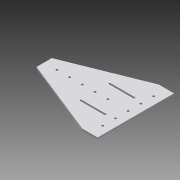
# Autodesk Inventor part: traingle_bracket(tb)
Saved by Autodesk Inventor 2015 (Build 190159000, 159)
## iProperties
Created: 2015-10-09
Part Number: traingle_bracket(tb)
Material: Aluminum 6061
Document SubType Name: Sheet Metal
Designer: elilitwack
Density: 2.7 g/cm^3
Sheet Metal Rule: Default
Appearance: Aluminum - Flat
Mass: 105.364 g
Surface Area: 274.012 cm^2
Volume: 39.0235 cm^3
Author: elilitwack
Autodesk Inventor part; units mm, degrees
ref_plane "YZ Plane" through (0, 0, 0) normal (1, 0, 0) x (0, 1, 0)
ref_plane "XZ Plane" through (0, 0, 0) normal (0, 1, 0) x (-1, 0, 0)
ref_plane "XY Plane" through (0, 0, 0) normal (0, 0, 1) x (1, 0, 0)
sketch "face_sketch" plane through (0, 0, 0) normal (0, 1, 0) x (-1, 0, 0)
  line L0 (0, 0) -> (25.4, 0)
  line L1 (25.4, 0) -> (25.4, -127)
  line L2 (25.4, -127) -> (0, -127)
  line L3 (0, -127) -> (0, 0)
  line L4 (25.4, -50.8) -> (152.4, -50.8)
  line L5 (152.4, -50.8) -> (152.4, -76.2)
  line L6 (152.4, -76.2) -> (25.4, -76.2)
  line L7 (25.4, -76.2) -> (25.4, -50.8)
  line L8 (152.4, -50.8) -> (25.4, 0)
  line L9 (152.4, -76.2) -> (25.4, -127)
  dimension "d0" = 25.4
  dimension "d1" = 127
  dimension "d2" = 127
  dimension "d3" = 25.4
  constraints: 20 end point, 4 parallel, 2 horizontal, 2 perpendicular, 1 equal length, 1 point on line
  measures "d0" distance of L1.end L2.end
  measures "d1" distance of L0.end L1.end
  measures "d2" distance of L5.end L6.end
  measures "d3" distance of L4.end L5.end
extrude "Plate1" add sketch "face_sketch" along normal blind 3.048
sketch "rivet_holes_sketch" plane through (0, 3.048, 0) normal (0, 1, 0) x (1, 0, 0)
  line L0 (-25.4, 0) -> (-152.4, 50.8) projected
  line L1 (0, 0) -> (-25.4, 0) projected
  line L2 (0, 127) -> (0, 0) projected
  line L3 (-25.4, 127) -> (0, 127) projected
  line L4 (-152.4, 76.2) -> (-25.4, 127) projected
  line L5 (-152.4, 50.8) -> (-152.4, 76.2) projected
  line L6 (-25.4, 127) -> (-25.4, 0) construction
  line L7 (0, 127) -> (-25.4, 127) construction
  line L8 (-25.4, 0) -> (0, 0) construction
  line L9 (-152.4, 76.2) -> (-152.4, 50.8) construction
  line L10 (-152.4, 63.5) -> (-131.2333, 63.5) construction
  line L11 (-131.2333, 63.5) -> (-110.0667, 63.5) construction
  line L12 (-110.0667, 63.5) -> (-88.9, 63.5) construction
  line L13 (-88.9, 63.5) -> (-67.7333, 63.5) construction
  line L14 (-67.7333, 63.5) -> (-46.5667, 63.5) construction
  line L15 (-46.5667, 63.5) -> (-25.4, 63.5) construction
  line L16 (-12.7, 0) -> (-12.7, 21.1667) construction
  line L17 (-12.7, 21.1667) -> (-12.7, 42.3333) construction
  line L18 (-12.7, 42.3333) -> (-12.7, 63.5) construction
  line L19 (-12.7, 63.5) -> (-12.7, 84.6667) construction
  line L20 (-12.7, 84.6667) -> (-12.7, 105.8333) construction
  line L21 (-12.7, 105.8333) -> (-12.7, 127) construction
  constraints: 26 end point, 10 coincident, 10 collinear, 8 point on line, 4 midpoint, 2 vertical, 1 horizontal
hole "rivet_holes" at (-131.2333, 3.048, -63.5) at (-110.0667, 3.048, -63.5) at (-88.9, 3.048, -63.5) at (-67.7333, 3.048, -63.5) at (-46.5667, 3.048, -63.5) at (-12.7, 3.048, -21.1667) at (-12.7, 3.048, -42.3333) at (-12.7, 3.048, -63.5) at (-12.7, 3.048, -84.6667) at (-12.7, 3.048, -105.8333) direction (0, -1, 0) diameter 3.5719 depth 3.048 tip angle 118
sketch "hm_mounting_slot_sketch" plane through (0, 3.048, 0) normal (0, 1, 0) x (1, 0, 0)
  line L0 (-67.437, 87.503) -> (-26.797, 87.503) construction
  line L1 (-67.437, 88.9) -> (-26.797, 88.9)
  line L2 (-26.797, 86.106) -> (-67.437, 86.106)
  arc A0 (-67.437, 88.9) -> (-67.437, 86.106) centre (-67.437, 87.503) ccw
  arc A1 (-26.797, 86.106) -> (-26.797, 88.9) centre (-26.797, 87.503) ccw
  line L3 (-67.437, 39.497) -> (-26.797, 39.497) construction
  line L4 (-67.437, 38.1) -> (-26.797, 38.1)
  line L5 (-26.797, 40.894) -> (-67.437, 40.894)
  arc A2 (-67.437, 40.894) -> (-67.437, 38.1) centre (-67.437, 39.497) ccw
  arc A3 (-26.797, 38.1) -> (-26.797, 40.894) centre (-26.797, 39.497) ccw
  line L6 (-25.4, 0) -> (-25.4, 127) construction
  line L7 (-68.834, 87.503) -> (-68.834, 109.6264) construction
  line L8 (-25.4, 127) -> (-152.4, 76.2) projected
  line L9 (-68.834, 39.497) -> (-68.834, 17.3736) construction
  line L10 (-152.4, 50.8) -> (-25.4, 0) projected
  point P0 (0, 0)
  point P1 (-47.117, 87.503)
  point P2 (-47.117, 39.497)
  point P3 (-25.4, 39.497)
  point P4 (-25.4, 87.503)
  point P5 (-68.834, 28.4353)
  dimension "d12" = 40.64
  dimension "d14" = 2.794
  dimension "d15" = 40.64
  dimension "d16" = 2.794
  dimension "d17" = 50.8
  constraints: 22 end point, 12 point on circle, 8 tangent, 4 centre point, 4 point on line, 3 midpoint, 3 vertical, 2 horizontal, 2 parallel, 1 collinear
  measures "d12" distance of L0.start L0.end
  measures "d14" distance between parallel lines of L2 L1
  measures "d15" distance of L3.start L3.end
  measures "d16" distance between parallel lines of L4 L5
  measures "d17" distance between parallel lines of L4 L1
extrude "Cut1" cut sketch "hm_mounting_slot_sketch" against normal blind 3.048
equation "\"d5\" = rv_hole_diameter"
equation "\"d10\" = Thickness"
equation "\"d12\" = tb_hm_mounting_slot_length"
equation "\"d15\" = tb_hm_mounting_slot_length"
equation "\"d17\" = hm_base_length"
equation "\"d18\" = Thickness"
equation "\"d0\" = st_outer_diameter"
equation "\"d1\" = tb_rivet_row_length"
equation "\"d2\" = tb_rivet_row_length"
equation "\"d3\" = st_outer_diameter"
equation "\"Thickness\" = tb_metal_thickness"
equation "\"BendRadius\" = Thickness"
equation "\"BendReliefWidth\" = Thickness"
equation "\"BendReliefDepth\" = 0.5 * Thickness"
equation "\"CornerReliefSize\" = 4 * Thickness"
equation "\"MinimumRemnant\" = 2 * Thickness"
equation "\"TransitionRadius\" = BendRadius"
equation "\"JacobiRadiusSize\" = BendRadius"
equation "\"GapSize\" = Thickness"
equation "\"bp_thickness\" = 3.048"
equation "\"bp_height\" = gb_mh_seperation + st_outer_diameter"
equation "\"bp_width\" = 4 * st_rivet_distance"
equation "\"bp_axle_height\" = magic_axle_offset + gb_axle_from_edge + gb_to_bottom_of_side_assembly"
equation "\"magic_axle_offset\" = 2.286"
equation "\"bp_tensioner_width\" = 6.35"
equation "\"bp_tensioner_height\" = 50.8"
equation "\"bp_tensioner_from_bottom\" = 38.1"
equation "\"bp_tensioner_from_side\" = 25.4"
equation "\"bp_tensioner_wood_mount_from_tensioner_top\" = 12.7"
equation "\"bp_tensioner_wood_mount_diameter\" = 6.35"
equation "\"gb_mh_seperation\" = 111.1504"
equation "\"gb_mh_diameter\" = 6.35"
equation "\"gb_axle_from_edge\" = 38.1"
equation "\"gb_width\" = 127"
equation "\"gb_bearing_diameter\" = 28.575"
equation "\"gb_to_bottom_of_side_assembly\" = 4.7752"
equation "\"rv_hole_diameter\" = 3.57187"
equation "\"st_outer_diameter\" = 25.4"
equation "\"st_wall_thickness\" = 1.5875"
equation "\"st_length\" = 685.8"
equation "\"st_gbmh_from_center\" = 0.5 * gb_mh_seperation"
equation "\"st_cutout_depth_right\" = 203.2"
equation "\"st_cutout_depth_left\" = 203.2"
equation "\"st_rivet_distance\" = 19.05"
equation "\"so_inner_diameter\" = 7.62"
equation "\"so_wall_thickness\" = 5.08"
equation "\"so_length\" = 40.64"
equation "\"twb_width\" = st_outer_diameter"
equation "\"twb_length\" = bp_tensioner_width + 2 * twb_margin_on_each_side"
equation "\"twb_height\" = 2 * bp_tensioner_wood_mount_diameter + bp_tensioner_height + 2 * bp_tensioner_wood_mount_from_tensioner_top + twb_margin_on_each_side"
equation "\"twb_margin_on_each_side\" = 6.35"
equation "\"twb_tensioner_from_edge\" = -0.5 * bp_tensioner_height + 0.5 * twb_height"
equation "\"tb_side_length\" = 127"
equation "\"tb_rivet_row_length\" = 127"
equation "\"d4\" = BendRadius"
equation "\"tb_metal_thickness\" = 3.048"
equation "\"tb_hm_mounting_slot_length\" = 40.64"
equation "\"hm_base_width\" = 30.48"
equation "\"hm_base_length\" = 50.8"
equation "\"hm_moon_flange_radius\" = 17.78"
equation "\"hm_moon_channel_offset\" = 2.286"
equation "\"hm_moon_flange_width\" = 5.08"
equation "\"hm_moon_thickness\" = 5.08"
equation "\"hm_base_height\" = 5.08"
equation "\"hm_peg_width\" = 2.54"
equation "\"hm_peg_length\" = 5.08"
equation "\"hm_peg_height\" = 5.08"
equation "\"hm_rivet_groove_width\" = 10.16"
equation "\"hm_rivet_groove_height\" = 1.27"
equation "\"gb_mh_seperation_alt\" = 111.125"
equation "\"gb_axle_from_edge_alt\" = 43.1546"
equation "\"bp_axle_height_alt\" = magic_axle_offset + gb_axle_from_edge_alt + gb_to_bottom_of_side_assembly"
body "Solid1"
